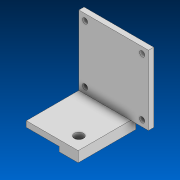
# Autodesk Inventor part: Battery Switch Mount
Saved by Autodesk Inventor 2022 (Build 260153000, 153)
## iProperties
Created: 2022-04-21
Part Number: Battery Switch Mount
Material: Generic
Document SubType Name: Modeling
Designer: score_nygvs6w
Density: 1 g/cm^3
Appearance: Default
Author: score_nygvs6w
Autodesk Inventor part; units mm, degrees
ref_plane "YZ Plane" through (0, 0, 0) normal (1, 0, 0) x (0, 1, 0)
ref_plane "XZ Plane" through (0, 0, 0) normal (0, 1, 0) x (-1, 0, 0)
ref_plane "XY Plane" through (0, 0, 0) normal (0, 0, 1) x (1, 0, 0)
sketch "Sketch1" plane through (0, 0, 0) normal (0, 0, 1) x (1, 0, 0)
  line L0 (33.655, 33.655) -> (-33.655, 33.655)
  line L1 (-33.655, 33.655) -> (-33.655, -33.655)
  line L2 (-33.655, -33.655) -> (33.655, -33.655)
  line L3 (33.655, -33.655) -> (33.655, 33.655)
  line L4 (33.655, 33.655) -> (-33.655, -33.655) construction
  line L5 (-33.655, 33.655) -> (33.655, -33.655) construction
  circle A0 centre (0, 0) radius 39.0641 construction
  point P0 (-27.6225, 27.6225)
  point P1 (27.6225, 27.6225)
  point P2 (27.6225, -27.6225)
  point P3 (-27.6225, -27.6225)
  dimension "d1" = 67.31
  dimension "d2" = 67.31
  dimension "d3" = 55.245
  constraints: 12 end point, 4 point on line, 2 horizontal alignment, 2 midpoint, 2 parallel, 2 vertical alignment, 1 coincident, 1 horizontal, 1 perpendicular, 3 other
  measures "d1" distance between parallel lines of L3 L1
  measures "d2" distance between parallel lines of L2 L0
  measures "d3" distance of point (27.622, 27.623) point (-27.623, 27.623)
extrude "Extrusion1" add sketch "Sketch1" along normal blind 5.08
hole "Hole1" at (-27.6225, 27.6225, 0) at (27.6225, 27.6225, 0) at (27.6225, -27.6225, 0) at (-27.6225, -27.6225, 0) direction (0, 0, 1) diameter 5.08 end through all
sketch "Sketch2" plane through (0, 0, 0) normal (0, 0, -1) x (-1, 0, 0)
  line L0 (33.655, -33.655) -> (-33.655, -33.655) projected
  line L1 (-16.51, -33.655) -> (-16.51, -43.815)
  line L2 (-16.51, -43.815) -> (1.905, -43.815)
  line L3 (1.905, -43.815) -> (1.905, -33.655)
  line L4 (-33.655, -33.655) -> (-33.655, 33.655) projected
  line L5 (1.905, -33.655) -> (1.905, -39.243)
  line L6 (1.905, -39.243) -> (33.655, -39.243)
  line L7 (33.655, -39.243) -> (33.655, -33.655)
  line L8 (33.655, 33.655) -> (33.655, -33.655) projected
  line L9 (33.655, -43.815) -> (-33.655, -43.815) construction
  point P0 (0, 0)
  dimension "d14" = 17.145
  dimension "d16" = 10.16
  dimension "d17" = 4.572
  dimension "d18" = 31.75
  constraints: 14 end point, 5 point on line, 2 collinear, 2 parallel, 1 horizontal
  measures "d14" distance between parallel lines of L1 L4
  measures "d16" distance between parallel lines of L0 L9
  measures "d17" distance between parallel lines of L6 L9
  measures "d18" distance between parallel lines of L7 L3
extrude "Extrusion2" add sketch "Sketch2" against normal blind 55.88
sketch "Sketch3" plane through (-1.905, -33.655, 0) normal (0, -1, 0) x (1, 0, 0)
  line L0 (0, 0) -> (0, 55.88) projected
  line L1 (0, 55.88) -> (18.415, 55.88) projected
  point P0 (1.905, 0)
  point P1 (6.35, 43.18)
  dimension "d21" = 6.35
  dimension "d22" = 12.7
  measures "d21" distance from line of L0 point (6.35, 43.18)
  measures "d22" distance from line of L1 point (6.35, 43.18)
hole "Hole2" at (4.445, -33.655, 43.18) direction (0, -1, 0) diameter 4.572 end through all counterbore diameter 8.89 counterbore depth 5.08
body "Solid1"
